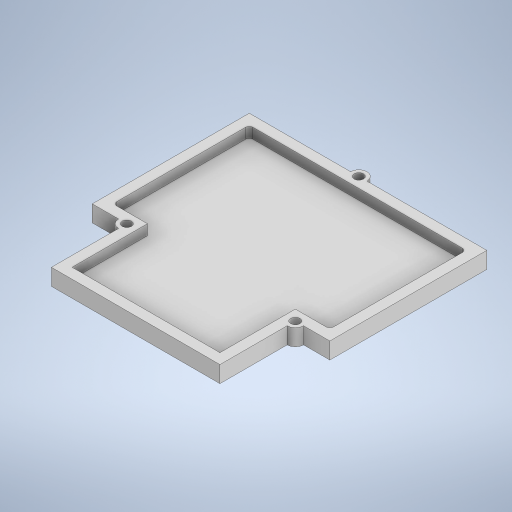
# Autodesk Inventor part: raspberry-coral-chasis-fastening
Saved by Autodesk Inventor 2024 (Build 280153000, 153)
## iProperties
Created: 2024-05-17
Part Number: raspberry-coral-chasis-fastening
Material: Generic
Document SubType Name: Modeling
Designer: inigo
Density: 1 g/cm^3
Appearance: Default
Author: inigo
Autodesk Inventor part; units mm, degrees
ref_plane "YZ Plane" through (0, 0, 0) normal (1, 0, 0) x (0, 1, 0)
ref_plane "XZ Plane" through (0, 0, 0) normal (0, 1, 0) x (-1, 0, 0)
ref_plane "XY Plane" through (0, 0, 0) normal (0, 0, 1) x (1, 0, 0)
sketch "Sketch1" plane through (0, 0, 0) normal (0, 1, 0) x (-1, 0, 0)
  line L0 (-40.2798, 52.2721) -> (31.3202, 52.2721)
  line L1 (-40.2798, 15.7721) -> (-40.2798, 52.2721)
  line L2 (-55.2966, 15.7721) -> (-40.2798, 15.7721)
  line L3 (-56.9798, 14.0889) -> (-56.9798, -48.5447)
  line L4 (46.337, -50.2279) -> (-55.2966, -50.2279)
  line L5 (48.0202, -24.2779) -> (48.0202, -48.5447)
  line L6 (48.0202, -9.7779) -> (48.0202, 14.0889)
  line L7 (31.3202, 15.7721) -> (46.337, 15.7721)
  line L8 (31.3202, 15.7721) -> (31.3202, 52.2721)
  line L9 (-56.784, 14.6914) -> (-56.9798, 14.0889)
  line L10 (-56.784, 14.6914) -> (-56.4116, 15.2039)
  line L11 (-55.2966, 15.7721) -> (-55.8991, 15.5763)
  line L12 (-56.4116, 15.2039) -> (-55.8991, 15.5763)
  spline S0 degree 4 poles (-56.9798, 14.0889) (-56.8811, 14.7163) (-56.5148, 15.3071) (-55.924, 15.6734) (-55.2966, 15.7721) knots 0 0 0 0 0 1 1 1 1 1
  line L13 (47.8244, 14.6914) -> (47.452, 15.2039)
  line L14 (46.337, 15.7721) -> (46.9395, 15.5763)
  line L15 (47.8244, 14.6914) -> (48.0202, 14.0889)
  line L16 (46.9395, 15.5763) -> (47.452, 15.2039)
  spline S1 degree 4 poles (46.337, 15.7721) (46.9644, 15.6734) (47.5552, 15.3071) (47.9215, 14.7163) (48.0202, 14.0889) knots 0 0 0 0 0 1 1 1 1 1
  line L17 (46.337, -50.2279) -> (46.9395, -50.0321)
  line L18 (47.452, -49.6597) -> (47.8244, -49.1472)
  line L19 (47.452, -49.6597) -> (46.9395, -50.0321)
  spline S2 degree 4 poles (48.0202, -48.5447) (47.9214, -49.1721) (47.5553, -49.763) (46.9644, -50.1292) (46.337, -50.2279) knots 0 0 0 0 0 1 1 1 1 1
  line L20 (-56.9798, -48.5447) -> (-56.784, -49.1472)
  line L21 (-55.2966, -50.2279) -> (-55.8991, -50.0321)
  spline S3 degree 4 poles (-55.2966, -50.2279) (-55.924, -50.1292) (-56.5149, -49.763) (-56.8811, -49.1721) (-56.9798, -48.5447) knots 0 0 0 0 0 1 1 1 1 1
  line L22 (48.0202, -9.7779) -> (48.0202, -24.2779)
  line L23 (-55.2966, 20.7721) -> (-45.2798, 20.7721)
  line L24 (-45.2798, 20.7721) -> (-45.2798, 57.2721)
  line L25 (-45.2798, 57.2721) -> (36.3202, 57.2721)
  line L26 (36.3202, 57.2721) -> (36.3202, 20.7721)
  line L27 (46.337, -55.2279) -> (-55.2966, -55.2279)
  line L28 (-61.9798, -48.5447) -> (-61.9798, 14.8809)
  line L29 (-45.2798, 20.7721) -> (-61.9798, 20.7721)
  line L30 (-61.9798, 20.7721) -> (-61.9798, -55.2279)
  line L31 (-61.9798, -55.2279) -> (53.0202, -55.2279)
  line L32 (53.0202, -55.2279) -> (53.0202, 20.7721)
  line L33 (53.0202, 20.7721) -> (36.3202, 20.7721)
  circle A0 centre (-45.2798, 20.7721) radius 2.25
  circle A1 centre (36.3202, 20.7721) radius 2.25
  circle A2 centre (0, -55.2279) radius 2.25
  circle A3 centre (36.3202, 20.7721) radius 4
  circle A4 centre (-45.2798, 20.7721) radius 4
  circle A5 centre (0, -55.2279) radius 4
  point P0 (0, 0)
  point P1 (32.0202, -45.2279)
  point P2 (-56.4116, -49.6597)
  point P3 (-56.4116, -49.6597)
  point P4 (40.3202, 20.7721)
  point P5 (36.3202, 24.7721)
  point P6 (-45.2798, 24.7721)
  point P7 (-49.2798, 20.7721)
  point P8 (-4, -55.2279)
  point P9 (4, -55.2279)
  point P10 (-56.9798, 14.0889)
  dimension "d0" = 5
  dimension "d2" = 5
  dimension "d3" = 5
  dimension "d4" = 4.5
  dimension "d5" = 4.5
  dimension "d6" = 4.5
  dimension "d7" = 8
  dimension "d8" = 8
  dimension "d9" = 8
  constraints: 68 end point, 6 centre point, 6 coincident, 3 perpendicular, 3 point on line, 1 collinear, 1 parallel, 23 other
  measures "d0" distance between parallel lines of L8 L26
  measures "d2" distance between parallel lines of L4 L27
  measures "d3" distance between parallel lines of L3 L28
  measures "d4" diameter of A0
  measures "d5" diameter of A1
  measures "d6" diameter of A2
  measures "d7" diameter of A3
  measures "d8" diameter of A4
  measures "d9" diameter of A5
extrude "Extrusion1" add sketch "Sketch1" along normal blind 5 contours L23 A4 L24 L25 L26 A3 L33 L32 L31 L27 A5 L30 L28 L29 | A4 L24 A0 L23 | L23 A0 L24 A4 | A3 L33 A1 L26 | L26 A1 L33 A3 | A5 L27 A2 | L27 A2 A5
sketch "Sketch2" plane through (0, 0, 0) normal (0, -1, 0) x (1, 0, 0)
  line L0 (61.9798, 20.7721) -> (61.9798, -55.2279) projected
  line L1 (49.2798, 20.7721) -> (61.9798, 20.7721) projected
  arc A0 (49.2798, 20.7721) -> (45.2798, 24.7721) centre (45.2798, 20.7721) ccw projected
  line L2 (45.2798, 57.2721) -> (45.2798, 24.7721) projected
  line L3 (-36.3202, 57.2721) -> (45.2798, 57.2721) projected
  line L4 (-36.3202, 24.7721) -> (-36.3202, 57.2721) projected
  arc A1 (-36.3202, 24.7721) -> (-40.3202, 20.7721) centre (-36.3202, 20.7721) ccw projected
  line L5 (-53.0202, 20.7721) -> (-40.3202, 20.7721) projected
  line L6 (-53.0202, -55.2279) -> (-53.0202, 20.7721) projected
  line L7 (-4, -55.2279) -> (-53.0202, -55.2279) projected
  arc A2 (-4, -55.2279) -> (4, -55.2279) centre (0, -55.2279) ccw projected
  line L8 (61.9798, -55.2279) -> (4, -55.2279) projected
  circle A3 centre (45.2798, 20.7721) radius 2.25 projected
  circle A4 centre (45.2798, 20.7721) radius 2.25
  circle A5 centre (0, -55.2279) radius 2.25
  circle A6 centre (-36.3202, 20.7721) radius 2.25
  point P0 (0, 0)
  constraints: 3 centre point, 3 coincident
extrude "Extrusion2" add sketch "Sketch2" along normal blind 3
body "Solid1"
